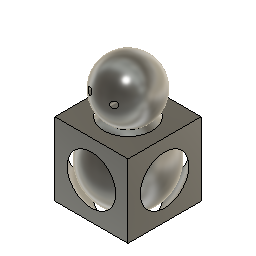
실기1 (Autodesk Fusion 360 design; units mm, degrees)
Autodesk Fusion 360 part; units mm, degrees
note: some values were not read from the file. Set by a fixed rule: which sketch regions a step uses.
sketch "Sketch2" plane through (0, 0, 0) normal (0, 1, 0) x (1, 0, 0)
  circle A0 centre (0, 0) radius 12
  line L0 (0, 0) -> (0, -25)
  circle A1 centre (0, -25) radius 9
  line L1 (0, -25) -> (0, -27)
  line L2 (0, -27) -> (-5, -27)
  circle A2 centre (-5, -27) radius 1.25
  circle A3 centre (5, -27) radius 1.25
  arc A4 (-6.2235, -14.74) -> (6.2235, -14.74) centre (0, -25) ccw
  line L3 (0, 14) -> (0, -37)
  line L4 (0, 0) -> (0, 14)
  line L5 (-7.746, 14) -> (7.746, 14)
  arc A5 (6.2235, -14.74) -> (7.746, 14) centre (0, 0) ccw
  arc A6 (-7.746, 14) -> (-6.2235, -14.74) centre (0, 0) ccw
  dimension "d2" = 32
  dimension "d3" = 24
  dimension "d4" = 25
  dimension "d5" = 24
  dimension "d6" = 18
  dimension "d7" = 2
  dimension "d8" = 5
  dimension "d9" = 2.5
  dimension "d13" = 14
  constraint coincident A0.centre L0.start
  constraint vertical L0
  constraint coincident L0.end A1.centre
  constraint parallel L0 L1
  constraint perpendicular L1 L2
  constraint coincident L2.end A2.centre
  constraint symmetric L1 A2 A3
  constraint midpoint A4 L3.end
  constraint parallel L3 L4
  constraint perpendicular L4 L5
  constraint concentric A5 A6
  measures "d2" diameter of A5
  measures "d3" diameter of A0
  measures "d4" distance of A0.centre L0.end
  measures "d5" diameter of A4
  measures "d6" diameter of A1
  measures "d7" distance of L0.end L1.end
  measures "d8" distance of L1.end L2.end
  measures "d9" diameter of A2
  measures "d13" distance of A0.centre L3.start
revolve "Revolve1" add sketch "Sketch2" angle 360 about axis through (0, 0, 0) along (0, 0, 1) contours A0 L0 A1 A4 L3 L4 L5 A6 makes body 1
extrude "Extrude1" cut sketch "Sketch2" against normal blind 33.921 contours A2 | A3 bodies 1
sketch "Sketch3" plane through (0, 0, 0) normal (0, 1, 0) x (1, 0, 0)
  line L0 (15, -15) -> (-15, -15)
  line L1 (-15, -15) -> (-15, 15)
  line L2 (-15, 15) -> (15, 15)
  line L3 (15, 15) -> (15, -15)
  line L4 (15, -15) -> (-15, 15) construction
  line L5 (-15, -15) -> (15, 15) construction
  circle A0 centre (0, 0) radius 18
  line L6 (0, 18) -> (0, -18)
  dimension "d14" = 30
  dimension "d15" = 30
  dimension "d16" = 36
  constraint perpendicular L0 L1
  constraint parallel L0 L2
  constraint parallel L1 L3
  constraint horizontal L0
  constraint coincident L4 A0.centre
  constraint coincident L5 A0.centre
  constraint coincident A0.centre origin
  constraint perpendicular L0 L6
  constraint coincident A0 L6.end
  constraint coincident A0 L6.start
  measures "d14" distance of L1.end L2.end
  measures "d15" distance of L0.end L1.end
  measures "d16" diameter of A0
extrude "Extrude2" add sketch "Sketch3" along normal mid plane 30 separate body contours L0 L3 A0 | L0 L2 L3 A0 L6 | L0 L1 L2 A0 L6 | L2 L3 A0 | L0 L1 A0 | L1 L2 A0 makes body 2
revolve "Revolve2" cut sketch "Sketch3" angle 360 about axis through (0, 0, -18) along (0, 0, 1) contours L0 A0 L6 | L0 L1 L2 A0 L6 | L2 A0 L6 | L1 A0 picked at (-0.8754, -16.9358) picked at (-0.8754, 16.9358) bodies 2
